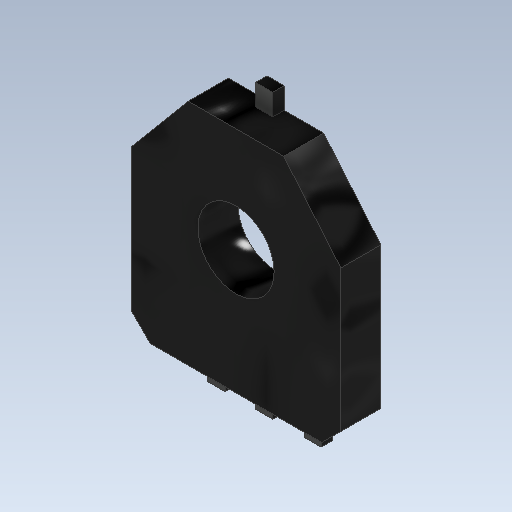
# Autodesk Inventor part: mainbody
Saved by Autodesk Inventor 2020 (Build 240168000, 168)
## iProperties
Created: 2020-01-18
Part Number: mainbody
Material: Generic
Document SubType Name: Modeling
Designer: sami_
Density: 1 g/cm^3
Appearance: Dark Gray
Author: sami_
Autodesk Inventor part; units mm, degrees
ref_plane "YZ Plane" through (0, 0, 0) normal (1, 0, 0) x (0, 1, 0)
ref_plane "XZ Plane" through (0, 0, 0) normal (0, 1, 0) x (-1, 0, 0)
ref_plane "XY Plane" through (0, 0, 0) normal (0, 0, 1) x (1, 0, 0)
sketch "Sketch1" plane through (0, 0, 0) normal (0, 0, 1) x (1, 0, 0)
  line L0 (10.2242, -22.1045) -> (46.869, -22.1045) construction
  line L1 (46.869, -22.1045) -> (46.869, -51.7203) construction
  line L2 (46.869, -51.7203) -> (10.2242, -51.7203) construction
  line L3 (10.2242, -51.7203) -> (10.2242, -22.1045) construction
  line L4 (29.8676, -31.4438) -> (29.8676, -43.4438) construction
  line L5 (33.8496, -35.029) -> (33.8496, -42.667)
  line L6 (33.8496, -42.667) -> (33.8496, -43.4438)
  line L7 (33.8496, -43.4438) -> (32.8496, -43.4438)
  line L8 (22.8496, -43.4438) -> (22.8496, -42.4438)
  line L9 (22.8496, -31.4438) -> (25.8496, -31.4438)
  line L10 (33.8496, -31.4438) -> (33.8496, -35.019)
  line L11 (28.3496, -31.4438) -> (28.3496, -43.4438) construction
  line L12 (28.3496, -31.4438) -> (25.8496, -31.4438)
  line L13 (25.8496, -31.4438) -> (22.8496, -35.019)
  line L14 (28.3496, -43.4438) -> (23.8496, -43.4438)
  line L15 (23.8496, -43.4438) -> (22.8496, -42.4438)
  line L16 (30.8496, -31.4438) -> (33.8496, -35.019)
  line L17 (32.8496, -43.4438) -> (33.8496, -42.4438)
  line L18 (25.8496, -31.4438) -> (30.8496, -31.4438)
  line L19 (22.8496, -35.019) -> (22.8496, -31.4438)
  line L20 (23.8496, -43.4438) -> (22.8496, -43.4438)
  line L21 (22.8496, -42.4438) -> (22.8496, -35.019)
  line L22 (32.8496, -43.4438) -> (23.8496, -43.4438)
  line L23 (33.8496, -43.4438) -> (33.8496, -43.6998)
  line L24 (33.8496, -42.4438) -> (33.8496, -43.4438)
  line L25 (33.8496, -35.019) -> (33.8496, -42.4438)
  line L26 (30.8496, -31.4438) -> (33.8496, -31.4438)
  circle A0 centre (28.3496, -36.9438) radius 2
  line L27 (26.6175, -35.9438) -> (30.0816, -35.9438)
  line L28 (25.0671, -43.4438) -> (25.3808, -43.8918)
  line L29 (25.0671, -43.4438) -> (25.614, -43.4438) construction
  line L30 (25.3808, -43.8918) -> (25.3808, -45.1736)
  line L31 (25.3808, -45.1736) -> (26.2783, -45.1736)
  line L32 (26.2783, -45.1736) -> (26.2783, -43.9789)
  line L33 (26.2783, -43.9789) -> (26.5414, -43.4438)
  line L34 (27.5656, -43.4438) -> (27.8793, -43.8918)
  line L35 (27.8793, -43.8918) -> (27.8793, -45.1736)
  line L36 (27.8793, -45.1736) -> (28.7769, -45.1736)
  line L37 (28.7769, -45.1736) -> (28.7769, -43.9789)
  line L38 (28.7769, -43.9789) -> (29.04, -43.4438)
  line L39 (31.6321, -43.4438) -> (31.3184, -43.8918)
  line L40 (31.3184, -43.8918) -> (31.3184, -45.1736)
  line L41 (31.3184, -45.1736) -> (30.4209, -45.1736)
  line L42 (30.4209, -45.1736) -> (30.4209, -43.9789)
  line L43 (30.4209, -43.9789) -> (30.1577, -43.4438)
  line L44 (31.6321, -43.4438) -> (31.3184, -43.8918)
  line L45 (31.3184, -43.8918) -> (31.3184, -45.1736)
  line L46 (31.3184, -45.1736) -> (30.4209, -45.1736)
  line L47 (30.4209, -45.1736) -> (30.4209, -43.9789)
  line L48 (30.4209, -43.9789) -> (30.1577, -43.4438)
  line L49 (31.6321, -43.4438) -> (31.3184, -43.8918)
  line L50 (31.3184, -43.8918) -> (31.3184, -45.1736)
  line L51 (31.3184, -45.1736) -> (30.4209, -45.1736)
  line L52 (30.4209, -45.1736) -> (30.4209, -43.9789)
  line L53 (30.4209, -43.9789) -> (30.1577, -43.4438)
  line L54 (28.7769, -30.3247) -> (27.8793, -30.3247)
  line L55 (27.8793, -30.3247) -> (27.8793, -31.4438)
  line L56 (27.8793, -31.4438) -> (28.7769, -31.4438)
  line L57 (28.7769, -31.4438) -> (28.7769, -30.3247)
  point P0 (0, 0)
  dimension "d1" = 12
  dimension "d57" = 11
  dimension "d58" = 2.5
  dimension "d59" = 130
  dimension "d60" = 4.5
  dimension "d61" = 135
  dimension "d66" = 4
  dimension "d69" = 6.5
  dimension "d70" = 3
  dimension "d71" = 55
  constraints: 108 end point, 20 parallel, 14 perpendicular, 10 symmetric about line, 6 horizontal, 6 point on line, 4 vertical, 2 point on circle, 1 centre point, 1 equal length, 2 other
  measures "d1" distance of L4.start L4.end
  measures "d57" distance of L9.start L10.start
  measures "d58" distance of L11.start L9.end
  measures "d59" angle of L13 L12
  measures "d60" distance of L11.end L14.end
  measures "d61" angle of L14 L15
  measures "d66" diameter of A0
  measures "d69" distance from line of L22 A0.centre
  measures "d71" angle of L28 L29
extrude "Extrusion1" add sketch "Sketch1" along normal blind 2.1 contours L5 L17 L22 L14 L15 L21 L13 L12 L18 L16 L25 | L39 L40 L41 L42 L43 L22 | L18 L12 L55 L54 L57 | L38 L37 L36 L35 L34 L14 L22 | L33 L32 L31 L30 L28 L14
sketch "Sketch2" plane through (0, 0, 2.1) normal (0, 0, 1) x (1, 0, 0)
  line L0 (23.8496, -43.4438) -> (25.0671, -43.4438) projected
  line L1 (25.0671, -43.4438) -> (32.3568, -43.4438)
  line L2 (32.3568, -43.4438) -> (32.3568, -45.6215)
  line L3 (32.3568, -45.6215) -> (25.0671, -45.6215)
  line L4 (25.0671, -45.6215) -> (25.0671, -43.4438)
  line L5 (27.8793, -30.3247) -> (27.8793, -31.4438) projected
  line L6 (28.7769, -31.4438) -> (28.7769, -30.3247) projected
  line L7 (27.8793, -31.4438) -> (28.7769, -31.4438)
  line L8 (28.7769, -31.4438) -> (28.7769, -30.3247)
  line L9 (28.7769, -30.3247) -> (27.8793, -30.3247)
  line L10 (27.8793, -30.3247) -> (27.8793, -31.4438)
  point P0 (0, 0)
  constraints: 16 end point, 4 parallel, 2 horizontal, 2 perpendicular
extrude "Extrusion2" cut sketch "Sketch2" against normal blind 1.5
body "Solid1"
